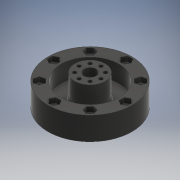
# Autodesk Inventor part: CS01
Saved by Autodesk Inventor 2017 (Build 210142000, 142)
## iProperties
Created: 2019-11-06
Part Number: CS01
Material: ABS Plastic
Document SubType Name: Modeling
Designer: Dell
Density: 1.06 g/cm^3
Appearance: Smooth - Black
Author: Dell
Autodesk Inventor part; units mm, degrees
ref_plane "YZ Plane" through (0, 0, 0) normal (1, 0, 0) x (0, 1, 0)
ref_plane "XZ Plane" through (0, 0, 0) normal (0, 1, 0) x (-1, 0, 0)
ref_plane "XY Plane" through (0, 0, 0) normal (0, 0, 1) x (1, 0, 0)
sketch "Sketch1" plane through (0, 0, 0) normal (0, 0, 1) x (1, 0, 0)
  circle A0 centre (0, 0) radius 5
  circle A1 centre (0, 0) radius 34.5
  dimension "d0" = 10
  dimension "d1" = 69
  constraints: 2 centre point, 2 coincident
  measures "d0" diameter of A0
  measures "d1" diameter of A1
extrude "Extrusion1" add sketch "Sketch1" along normal blind 5
sketch "Sketch2" plane through (0, 0, 5) normal (0, 0, 1) x (1, 0, 0)
  circle A0 centre (0, 0) radius 24
  circle A1 centre (0, 0) radius 34.5 projected
  dimension "d4" = 48
  constraints: 1 centre point, 1 coincident
  measures "d4" diameter of A0
extrude "Extrusion2" add sketch "Sketch2" along normal blind 14
sketch "Sketch3" plane through (0, 0, 5) normal (0, 0, 1) x (1, 0, 0)
  circle A0 centre (0, 0) radius 12.5
  circle A1 centre (0, 0) radius 5 projected
  dimension "d7" = 25
  constraints: 1 centre point, 1 coincident
  measures "d7" diameter of A0
extrude "Extrusion3" add sketch "Sketch3" along normal blind 20
chamfer "Chamfer1" distance 4 angle 15 1 edges at (-12.5, 0, 5) measured on face at (-12.5, 0, 5.5)
sketch "Sketch4" plane through (0, 0, 25) normal (0, 0, 1) x (1, 0, 0)
  circle A0 centre (9, 0) radius 1.5
  circle A1 centre (6.364, 6.364) radius 1.5
  circle A2 centre (0, 9) radius 1.5
  circle A3 centre (-6.364, 6.364) radius 1.5
  circle A4 centre (-9, 0) radius 1.5
  circle A5 centre (-6.364, -6.364) radius 1.5
  circle A6 centre (0, -9) radius 1.5
  circle A7 centre (6.364, -6.364) radius 1.5
  point P0 (0, 0)
  dimension "d13" = 3
  dimension "d14" = 9
  dimension "d17" = 360
  constraints: 8 centre point, 1 horizontal alignment, 17 other
  measures "d13" diameter of A0
  measures "d14" distance of A0.centre point (0, 0)
extrude "Extrusion4" cut sketch "Sketch4" against normal through all
sketch "Sketch5" plane through (0, 0, 19) normal (0, 0, 1) x (1, 0, 0)
  circle A0 centre (29.5, 0) radius 2
  circle A1 centre (20.8597, 20.8597) radius 2
  circle A2 centre (0, 29.5) radius 2
  circle A3 centre (-20.8597, 20.8597) radius 2
  circle A4 centre (-29.5, 0) radius 2
  circle A5 centre (-20.8597, -20.8597) radius 2
  circle A6 centre (0, -29.5) radius 2
  circle A7 centre (20.8597, -20.8597) radius 2
  point P0 (0, 0)
  dimension "d21" = 4
  dimension "d22" = 29.5
  dimension "d25" = 360
  constraints: 8 centre point, 1 horizontal alignment, 17 other
  measures "d21" diameter of A0
  measures "d22" distance of point (0, 0) A0.centre
extrude "Extrusion5" cut sketch "Sketch5" against normal through all
sketch "Sketch7" plane through (0, 0, 0) normal (0, 0, -1) x (-1, 0, 0)
  circle A0 centre (0, 9) radius 1.5 projected
  circle A1 centre (0, 9) radius 6.5
  circle A2 centre (0, 0) radius 15.5
  dimension "d29" = 13
  constraints: 2 centre point, 2 coincident, 1 tangent
  measures "d29" diameter of A1
extrude "Extrusion6" cut sketch "Sketch7" against normal blind 3 contours A0 | A1 | A2
sketch "Sketch8" plane through (0, 0, 19) normal (0, 0, 1) x (1, 0, 0)
  circle A0 centre (29.5, 0) radius 2 projected
  circle A1 centre (29.5, 0) radius 2 projected
  line L0 (29.5, 4.3301) -> (33.25, 2.1651)
  line L1 (33.25, 2.1651) -> (33.25, -2.1651)
  line L2 (33.25, -2.1651) -> (29.5, -4.3301)
  line L3 (29.5, -4.3301) -> (25.75, -2.1651)
  line L4 (25.75, -2.1651) -> (25.75, 2.1651)
  line L5 (25.75, 2.1651) -> (29.5, 4.3301)
  line L6 (17.7978, 23.9215) -> (21.9804, 25.0422)
  line L7 (21.9804, 25.0422) -> (25.0422, 21.9804)
  line L8 (25.0422, 21.9804) -> (23.9215, 17.7978)
  line L9 (23.9215, 17.7978) -> (19.7389, 16.6771)
  line L10 (19.7389, 16.6771) -> (16.6771, 19.7389)
  line L11 (16.6771, 19.7389) -> (17.7978, 23.9215)
  line L12 (-4.3301, 29.5) -> (-2.1651, 33.25)
  line L13 (-2.1651, 33.25) -> (2.1651, 33.25)
  line L14 (2.1651, 33.25) -> (4.3301, 29.5)
  line L15 (4.3301, 29.5) -> (2.1651, 25.75)
  line L16 (2.1651, 25.75) -> (-2.1651, 25.75)
  line L17 (-2.1651, 25.75) -> (-4.3301, 29.5)
  line L18 (-23.9215, 17.7978) -> (-25.0422, 21.9804)
  line L19 (-25.0422, 21.9804) -> (-21.9804, 25.0422)
  line L20 (-21.9804, 25.0422) -> (-17.7978, 23.9215)
  line L21 (-17.7978, 23.9215) -> (-16.6771, 19.7389)
  line L22 (-16.6771, 19.7389) -> (-19.7389, 16.6771)
  line L23 (-19.7389, 16.6771) -> (-23.9215, 17.7978)
  line L24 (-29.5, -4.3301) -> (-33.25, -2.1651)
  line L25 (-33.25, -2.1651) -> (-33.25, 2.1651)
  line L26 (-33.25, 2.1651) -> (-29.5, 4.3301)
  line L27 (-29.5, 4.3301) -> (-25.75, 2.1651)
  line L28 (-25.75, 2.1651) -> (-25.75, -2.1651)
  line L29 (-25.75, -2.1651) -> (-29.5, -4.3301)
  line L30 (-17.7978, -23.9215) -> (-21.9804, -25.0422)
  line L31 (-21.9804, -25.0422) -> (-25.0422, -21.9804)
  line L32 (-25.0422, -21.9804) -> (-23.9215, -17.7978)
  line L33 (-23.9215, -17.7978) -> (-19.7389, -16.6771)
  line L34 (-19.7389, -16.6771) -> (-16.6771, -19.7389)
  line L35 (-16.6771, -19.7389) -> (-17.7978, -23.9215)
  line L36 (4.3301, -29.5) -> (2.1651, -33.25)
  line L37 (2.1651, -33.25) -> (-2.1651, -33.25)
  line L38 (-2.1651, -33.25) -> (-4.3301, -29.5)
  line L39 (-4.3301, -29.5) -> (-2.1651, -25.75)
  line L40 (-2.1651, -25.75) -> (2.1651, -25.75)
  line L41 (2.1651, -25.75) -> (4.3301, -29.5)
  line L42 (23.9215, -17.7978) -> (25.0422, -21.9804)
  line L43 (25.0422, -21.9804) -> (21.9804, -25.0422)
  line L44 (21.9804, -25.0422) -> (17.7978, -23.9215)
  line L45 (17.7978, -23.9215) -> (16.6771, -19.7389)
  line L46 (16.6771, -19.7389) -> (19.7389, -16.6771)
  line L47 (19.7389, -16.6771) -> (23.9215, -17.7978)
  point P0 (0, 0)
  point P1 (20.8597, 20.8597)
  point P2 (0, 29.5)
  point P3 (-20.8597, 20.8597)
  point P4 (-29.5, 0)
  point P5 (-20.8597, -20.8597)
  point P6 (0, -29.5)
  point P7 (20.8597, -20.8597)
  dimension "d32" = 7.5
  dimension "d35" = 360
  constraints: 96 end point, 1 coincident, 1 vertical, 118 other
  measures "d32" distance between parallel lines of L1 L4
extrude "Extrusion7" cut sketch "Sketch8" against normal blind 4 contours A0 | L0 L1 L2 L3 L4 L5 | L6 L7 L8 L9 L10 L11 | L12 L13 L14 L15 L16 L17 | L18 L19 L20 L21 L22 L23 | L24 L25 L26 L27 L28 L29 | L30 L31 L32 L33 L34 L35 | L36 L37 L38 L39 L40 L41 | L42 L43 L44 L45 L46 L47
body "Solid1"
